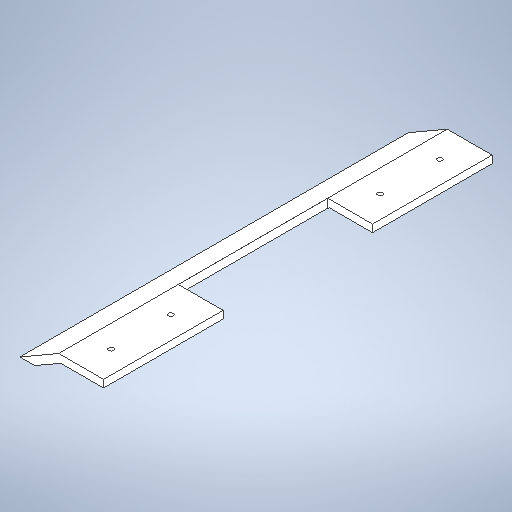
# Autodesk Inventor part: バンパー
Saved by Autodesk Inventor 2026.2 (Build 302298010, 298A)
## iProperties
Created: 2026-05-06
Part Number: バンパー
Material: 一般
Document SubType Name: Modeling
Designer: Yagis
Density: 1 g/cm^3
Appearance: 既定
Author: Yagis
Autodesk Inventor part; units mm, degrees
ref_plane "YZ Plane" through (0, 0, 0) normal (1, 0, 0) x (0, 1, 0)
ref_plane "XZ Plane" through (0, 0, 0) normal (0, 1, 0) x (-1, 0, 0)
ref_plane "XY Plane" through (0, 0, 0) normal (0, 0, 1) x (1, 0, 0)
sketch "スケッチ1" plane through (0, 0, 0) normal (0, 0, 1) x (1, 0, 0)
  line L0 (0, 0) -> (25.9808, 15)
  line L1 (25.9808, 15) -> (55.9808, 15)
  line L2 (55.9808, 15) -> (55.9808, 10)
  line L3 (55.9808, 10) -> (27.3205, 10)
  line L4 (27.3205, 10) -> (10, 0)
  line L5 (10, 0) -> (0, 0)
  dimension "d0" = 15
  dimension "d1" = 5
  dimension "d2" = 5
  dimension "d3" = 30
  dimension "d21" = 30
  constraints: 12 end point, 2 horizontal, 2 perpendicular, 1 parallel
  measures "d0" vertical distance of L0.start L0.end
  measures "d1" distance between parallel lines of L3 L1
  measures "d2" distance between parallel lines of L4 L0
  measures "d3" angle of L5 L4
  measures "d21" distance of L0.end L1.end
extrude "押し出し1" add sketch "スケッチ1" along normal blind 260
sketch "スケッチ2" plane through (25.9808, 15, 0) normal (0, 1, 0) x (1, 0, 0)
  line L0 (0.0508, -80) -> (34.0508, -80)
  line L1 (34.0508, -80) -> (34.0508, -180)
  line L2 (34.0508, -180) -> (0.0508, -180)
  line L3 (0.0508, -180) -> (0.0508, -80)
  line L4 (30, 0) -> (0, 0) projected
  line L5 (30, -260) -> (0, -260) projected
  point P0 (-25.9808, 0)
  point P1 (15, 0)
  point P2 (17.0508, -180)
  point P3 (15, -260)
  dimension "d7" = 80
  dimension "d8" = 80
  dimension "d22" = 34
  constraints: 8 end point, 3 midpoint, 2 parallel, 1 horizontal, 1 perpendicular
  measures "d7" distance between parallel lines of L0 L4
  measures "d8" vertical distance of point (17.051, -180) point (15, -260)
  measures "d22" distance between parallel lines of L3 L1
extrude "押し出し2" cut sketch "スケッチ2" against normal blind 300
sketch "スケッチ3" plane through (25.9808, 15, 0) normal (0, 1, 0) x (1, 0, 0)
  line L0 (30, 0) -> (30, -260) projected
  line L1 (30, 0) -> (0, 0) projected
  line L2 (30, -260) -> (0, -260) projected
  point P0 (-25.9808, 0)
  point P1 (15, -20)
  point P2 (15, -200)
  point P3 (30, -80)
  point P4 (15, -60)
  point P5 (15, -240)
  point P6 (15, -260)
  dimension "d12" = 15
  dimension "d13" = 20
  dimension "d23" = 40
  dimension "d24" = 20
  dimension "d25" = 40
  constraints: 3 vertical alignment, 1 midpoint
  measures "d12" distance from line of point (15, -20) L0
  measures "d13" distance from line of point (15, -20) L1
  measures "d23" distance of point (15, -60) point (15, -20)
  measures "d24" distance of point (15, -240) point (15, -260)
  measures "d25" distance of point (15, -240) point (15, -200)
hole "穴1" at (40.9808, 15, 20) at (40.9808, 15, 200) at (40.9808, 15, 60) at (40.9808, 15, 240) direction (0, -1, 0) diameter 3.2 depth 10 tip angle 118
